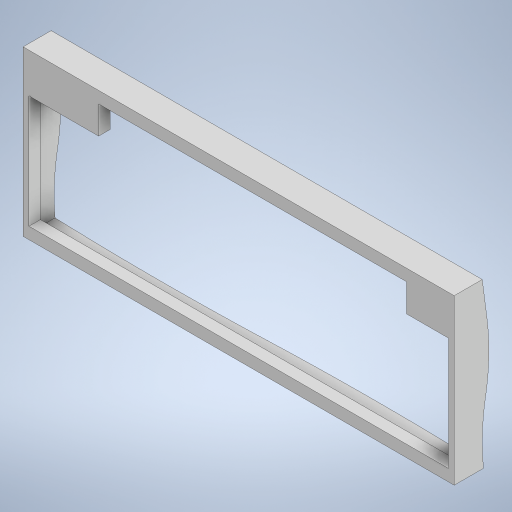
# Autodesk Inventor part: top
Saved by Autodesk Inventor 2024.2 (Build 282272000, 272)
## iProperties
Created: 2024-07-29
Part Number: top
Material: Generic
Document SubType Name: Modeling
Designer: Eric
Density: 1 g/cm^3
Appearance: Default
Author: Eric
Autodesk Inventor part; units mm, degrees
ref_plane "YZ Plane" through (0, 0, 0) normal (1, 0, 0) x (0, 1, 0)
ref_plane "XZ Plane" through (0, 0, 0) normal (0, 1, 0) x (-1, 0, 0)
ref_plane "XY Plane" through (0, 0, 0) normal (0, 0, 1) x (1, 0, 0)
ref_plane "Work Plane1" through (0, 0, 0) normal (0, 0, 1) x (1, 0, 0)
sketch "Sketch1" plane through (0, 0, 0) normal (0, 0, 1) x (1, 0, 0)
  line L0 (143.35, -48.1) -> (143.35, 29.05)
  line L1 (143.35, 29.05) -> (114.775, 29.05)
  line L2 (114.775, 29.05) -> (114.775, 48.1)
  line L3 (114.775, 48.1) -> (-95.725, 48.1)
  line L4 (-95.725, 48.1) -> (-95.725, 29.05)
  line L5 (-95.725, 29.05) -> (-143.35, 29.05)
  line L6 (-143.35, 29.05) -> (-143.35, -48.1)
  line L7 (-143.35, -48.1) -> (143.35, -48.1)
  line L8 (147.35, -56.1) -> (-147.35, -56.1)
  line L9 (-147.35, -56.1) -> (-147.35, 56.1)
  line L10 (-147.35, 56.1) -> (147.35, 56.1)
  line L11 (147.35, 56.1) -> (147.35, -56.1)
  line L12 (140.35, -31.6) -> (140.35, -44.6)
  line L13 (139.85, -45.1) -> (126.85, -45.1)
  line L14 (-140.35, -44.6) -> (-140.35, -31.6)
  line L15 (-92.725, 31.6) -> (-92.725, 44.6)
  line L16 (111.775, 44.6) -> (111.775, 31.6)
  line L17 (98.275, 45.1) -> (111.275, 45.1)
  line L18 (114.9437, 26.05) -> (127.9437, 26.05)
  point P0 (0, 0)
extrude "Extrusion1" add sketch "Sketch1" along normal blind 7.8
sketch "Sketch2" plane through (-147.35, -56.1, 0) normal (-1, 0, 0) x (0, 0, 1)
  line L0 (0, 112.2) -> (0, 0) projected
  line L1 (0, 112.2) -> (-11.364, 112.2)
  line L2 (0, 112.2) -> (7.8, 112.2) projected
  line L3 (-11.364, 112.2) -> (-14.6271, 87.4139)
  arc A0 (-14.6271, 87.4139) -> (-13.6566, 41.9302) centre (134.0896, 67.8349) ccw
  arc A1 (-11.9457, 3.275) -> (-13.6566, 41.9302) centre (-161.4028, 16.0255) ccw
  arc A2 (-11.9457, 3.275) -> (-12, 2) centre (3, 2) ccw
  line L4 (-12, 2) -> (-12, 0)
  line L5 (0, 0) -> (-12, 0)
  line L6 (0, 0) -> (7.8, 0) projected
  line L7 (-11.364, 112.2) -> (-11.0375, 114.68) construction
  line L8 (7.8, 112.2) -> (-11.0375, 114.68) construction
  point P0 (0, 56.1)
  dimension "d14" = 97.5
  dimension "d15" = 25
  dimension "d16" = 150
  dimension "d17" = 150
  dimension "d18" = 2
  dimension "d19" = 15
  dimension "d22" = 12
  dimension "d34" = 19
  dimension "d35" = 19.1639
  constraints: 12 end point, 6 point on circle, 4 tangent, 3 centre point, 3 perpendicular, 1 collinear, 1 horizontal
  measures "d14" angle of L3 L1
  measures "d15" distance of L1.end L3.end
  measures "d16" radius of A0
  measures "d17" radius of A1
  measures "d18" distance of L4.start L4.end
  measures "d19" radius of A2
  measures "d22" distance of L0.end L4.end
  measures "d34" distance of L2.end L7.end
  measures "d35" distance of L2.end L1.end
extrude "Extrusion2" add sketch "Sketch2" against normal blind 2
mirror "Mirror1" about plane through (0, 0, 0) normal (1, 0, 0) of "Extrusion2"
sketch "Sketch3" plane through (0, 0, 0) normal (0, 0, -1) x (-1, 0, 0)
  line L0 (-145.35, 56.1) -> (145.35, 56.1) projected
  line L1 (145.35, -56.1) -> (-145.35, -56.1) projected
  line L2 (145.35, -56.1) -> (145.35, 56.1) projected
  line L3 (-145.35, 56.1) -> (-145.35, -56.1) projected
  line L4 (145.35, 54.1) -> (-145.35, 54.1)
  line L5 (145.35, -54.1) -> (-145.35, -54.1)
  point P0 (0, 0)
  dimension "d25" = 2
  dimension "d26" = 2
  constraints: 4 end point, 4 point on line, 2 perpendicular
  measures "d25" distance between parallel lines of L4 L0
  measures "d26" distance between parallel lines of L1 L5
extrude "Extrusion3" add sketch "Sketch3" along normal up to surface contours L0 L2 L4 L3 surface through (-147.35, 31.3139, -14.6271) normal (0, 0.1305262, -0.9914449)
sketch "Sketch4" plane through (-147.35, -56.1, 7.8) normal (0, -1, 0) x (1, 0, 0)
  line L0 (2, -7.8) -> (2, -19.8) projected
  line L1 (2, -7.8) -> (292.7, -7.8) projected
  line L2 (292.7, -7.8) -> (292.7, -19.8) projected
  line L3 (0, -19.8) -> (2, -19.8) projected
  line L4 (294.7, -19.8) -> (292.7, -19.8) projected
  arc A0 (2, -19.8) -> (2.542, -19.7902) centre (2, -4.8) ccw
  arc A1 (147.35, -19.8) -> (2.542, -19.7902) centre (74.8108, -2018.4841) ccw
  arc A2 (147.35, -19.8) -> (292.158, -19.8098) centre (219.8892, 1978.8841) ccw
  arc A3 (292.7, -19.8) -> (292.158, -19.8098) centre (292.7, -34.8) ccw
  point P0 (147.35, -7.8)
  point P1 (147.35, -7.8)
  dimension "d29" = 15
  dimension "d30" = 2000
  dimension "d36" = 2000
  constraints: 8 point on circle, 5 tangent, 4 centre point, 1 equal radius, 1 midpoint, 1 vertical alignment
  measures "d29" radius of A0
  measures "d30" radius of A1
  measures "d36" radius of A2
extrude "Extrusion4" add sketch "Sketch4" against normal blind 2
body "Solid1"
